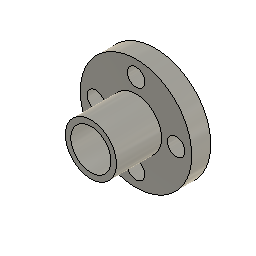
1dda108f-e19c-4853-9f5d-9e5fe5949c97 (Autodesk Fusion 360 design; units mm, degrees)
Autodesk Fusion 360 part; units mm, degrees
note: some values were not read from the file. Set by a fixed rule: which sketch regions a step uses.
sketch "Sketch1" plane through (0, 0, 0) normal (0, 1, 0) x (1, 0, 0)
  circle A0 centre (0, 0) radius 11.1
  dimension "d1" = 22.2
  measures "d1" diameter of A0
extrude "Extrude1" add sketch "Sketch1" along normal blind 3.8
sketch "Sketch2" plane through (0, 0, 0) normal (0, -1, 0) x (1, 0, 0)
  circle A0 centre (0, 0) radius 11.1
  circle A1 centre (0, 0) radius 5.1
  dimension "d4" = 10.2
  measures "d4" diameter of A1
extrude "Extrude2" add sketch "Sketch2" along normal blind 9 contours A1
sketch "Sketch3" plane through (0, 3.8, 0) normal (0, 1, 0) x (-1, 0, 0)
  circle A0 centre (0, 0) radius 11.1
  circle A1 centre (0, 0) radius 5.1
  dimension "d7" = 10.2
  measures "d7" diameter of A1
extrude "Extrude3" add sketch "Sketch3" along normal blind 2 contours A1
sketch "Sketch4" plane through (0, 5.8, 0) normal (0, 1, 0) x (-1, 0, 0)
  circle A0 centre (0, 0) radius 5.1
  circle A1 centre (0, 0) radius 4
  dimension "d10" = 8
  measures "d10" diameter of A1
extrude "Extrude4" cut sketch "Sketch4" against normal blind 17 contours A1
sketch "Sketch5" plane through (0, 0, 0) normal (0, -1, 0) x (1, 0, 0)
  circle A0 centre (0, 0) radius 5.1
  circle A1 centre (0, 0) radius 11.1
  circle A2 centre (0, 0) radius 8
  circle A3 centre (-8, 0) radius 1.75
  line L0 (0, 0) -> (-16, 0)
  line L1 (-16, 0) -> (-16, 13)
  line L2 (-16, 13) -> (0, 13)
  line L3 (0, 13) -> (0, 0)
  line L4 (0, 0) -> (14, 0)
  line L5 (14, 0) -> (14, -12)
  line L6 (14, -12) -> (0, -12)
  line L7 (0, -12) -> (0, 0)
  circle A4 centre (0, 8) radius 1.75
  circle A5 centre (0, -8) radius 1.75
  circle A6 centre (8, 0) radius 1.75
  dimension "d13" = 16
  dimension "d14" = 3.5
  dimension "d15" = 3.5
  dimension "d16" = 3.5
  dimension "d17" = 3.5
  measures "d13" diameter of A2
  measures "d14" diameter of A3
  measures "d15" diameter of A4
  measures "d16" diameter of A5
  measures "d17" diameter of A6
extrude "Extrude5" cut sketch "Sketch5" against normal blind 7 contours A2 L4 A6 | A2 L4 A6 | A2 L3 A4 | A2 L3 A4 | A2 L7 A5 | A2 L7 A5 | A2 L4 A6 | A2 L4 A6 | A2 A3 L0 | A2 A3 L0 | A2 L3 A4 | A2 L3 A4 | A2 L7 A5 | A2 L7 A5 | A2 A3 L0 | A2 A3 L0
